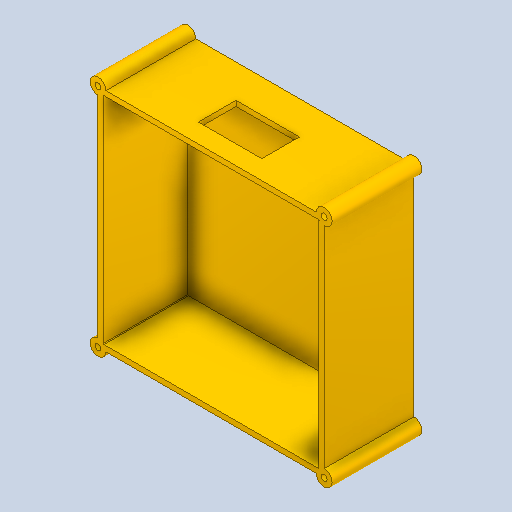
# Autodesk Inventor part: PS-01
Saved by Autodesk Inventor 2022 (Build 260153000, 153)
## iProperties
Company: El Camino College
Created: 2023-06-09
Part Number: PS-01
Material: Aluminum 6061(1)
Document SubType Name: Modeling
Designer: Edgar Tejada
Density: 2.7 g/cm^3
Appearance: Aluminum - Flat(1)
Mass: 407.53 g
Surface Area: 967.957 cm^2
Volume: 150.937 cm^3
Description: Aluminum Panel Cover
Author: Edgar Tejada
Title: Panel Shell
Autodesk Inventor part; units mm, degrees
ref_plane "YZ Plane" through (0, 0, 0) normal (1, 0, 0) x (0, 1, 0)
ref_plane "XZ Plane" through (0, 0, 0) normal (0, 1, 0) x (-1, 0, 0)
ref_plane "XY Plane" through (0, 0, 0) normal (0, 0, 1) x (1, 0, 0)
sketch "Sketch1" plane through (0, 0, 0) normal (0, 0, 1) x (1, 0, 0)
  line L0 (-64.77, 64.77) -> (64.77, 64.77)
  line L1 (64.77, 64.77) -> (64.77, -64.77)
  line L2 (64.77, -64.77) -> (-64.77, -64.77)
  line L3 (-64.77, -64.77) -> (-64.77, 64.77)
  line L4 (-64.77, 64.77) -> (64.77, -64.77) construction
  line L5 (64.77, 64.77) -> (-64.77, -64.77) construction
  point P0 (0, 0)
  dimension "d0" = 129.54
  constraints: 12 end point, 2 midpoint, 2 parallel, 2 perpendicular, 1 horizontal
  measures "d0" distance of L2.end L0.start
extrude "Extrusion1" add sketch "Sketch1" along normal blind 50.8
shell "Shell1" thickness 3.175 outward yes removed faces 1 at (-21.59, -21.59, 50.8)
sketch "Sketch2" plane through (0, 0, 0) normal (0, 0, 1) x (1, 0, 0)
  line L0 (-67.945, 67.945) -> (-67.945, -67.945) projected
  circle A0 centre (-67.945, 67.945) radius 4.7752
  line L1 (67.945, -67.945) -> (67.945, 67.945) projected
  circle A1 centre (67.945, 67.945) radius 4.7752
  line L2 (-67.945, -67.945) -> (67.945, -67.945) projected
  circle A2 centre (67.945, -67.945) radius 4.7752
  circle A3 centre (-67.945, -67.945) radius 4.7752
  point P0 (0, 0)
  dimension "d4" = 9.5504
  constraints: 4 centre point, 3 equal radius, 2 coincident
  measures "d4" diameter of A0
extrude "Extrusion2" add sketch "Sketch2" along normal blind 50.8 and the other way blind 3.175
sketch "Sketch3" plane through (0, 0, 50.8) normal (0, 0, 1) x (1, 0, 0)
  line L0 (-67.945, 63.1698) -> (-67.945, -63.1698) projected
  circle A0 centre (-67.945, -67.945) radius 1.7996
  line L1 (-63.1698, -67.945) -> (63.1698, -67.945) projected
  arc A1 (-67.945, -63.1698) -> (-63.1698, -67.945) centre (-67.945, -67.945) ccw projected
  arc A2 (-63.1698, 67.945) -> (-67.945, 63.1698) centre (-67.945, 67.945) ccw projected
  circle A3 centre (-67.945, 67.945) radius 1.7996
  arc A4 (67.945, 63.1698) -> (63.1698, 67.945) centre (67.945, 67.945) ccw projected
  circle A5 centre (67.945, 67.945) radius 1.7996
  arc A6 (63.1698, -67.945) -> (67.945, -63.1698) centre (67.945, -67.945) ccw projected
  circle A7 centre (67.945, -67.945) radius 1.7996
  point P0 (0, 0)
  point P1 (82.55, 82.55)
  dimension "d17" = 3.5992
  constraints: 4 centre point, 3 coincident, 3 equal radius, 1 concentric
  measures "d17" diameter of A0
extrude "Extrusion3" cut sketch "Sketch3" along normal mid plane 107.95
sketch "Sketch4" plane through (-63.1698, 67.945, -3.175) normal (0, 1, 0) x (1, 0, 0)
  line L0 (44.1198, -19.939) -> (82.2198, -19.939)
  line L1 (82.2198, -19.939) -> (82.2198, -42.545)
  line L2 (82.2198, -42.545) -> (44.1198, -42.545)
  line L3 (44.1198, -42.545) -> (44.1198, -19.939)
  line L4 (44.1198, -19.939) -> (82.2198, -42.545) construction
  line L5 (82.2198, -19.939) -> (44.1198, -42.545) construction
  line L6 (126.3396, -53.975) -> (0, -53.975) projected
  point P0 (63.1698, -3.175)
  point P1 (63.1698, -31.242)
  point P2 (63.1698, -31.242)
  point P3 (160.9128, -53.975)
  point P4 (-0.588, -53.975)
  dimension "d12" = 38.1
  dimension "d13" = 22.606
  dimension "d14" = 11.43
  constraints: 12 end point, 3 midpoint, 2 parallel, 1 horizontal, 1 perpendicular, 1 vertical alignment
  measures "d12" distance of L0.start L0.end
  measures "d13" distance of L0.end L1.end
  measures "d14" distance between parallel lines of L2 L6
extrude "Extrusion4" cut sketch "Sketch4" against normal up to next
body "Solid1"
